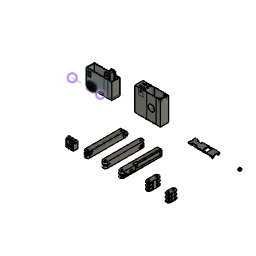
Table Lamp 2.0 v49 (Autodesk Fusion 360 design; units mm, degrees)
Autodesk Fusion 360 part; units mm, degrees
(part 1 of 2)
sketch "Schizzo1" plane through (0, 0, 0) normal (0, 0, 1) x (1, 0, 0)
  line L0 (0, 0) -> (100, 0)
  line L1 (100, 0) -> (100, 150)
  line L2 (100, 150) -> (0, 150)
  line L3 (0, 150) -> (0, 0)
  line L4 (199.5017, -0.6) -> (225.5017, -0.6)
  line L5 (225.5017, -0.6) -> (225.5017, 15.4)
  line L6 (225.5017, 15.4) -> (199.5017, 15.4)
  line L7 (199.5017, 15.4) -> (199.5017, -0.6)
  line L8 (212.5017, 15.4) -> (212.5017, -0.6) construction
  line L9 (199.5017, 7.4) -> (225.5017, 7.4) construction
  line L10 (199.5017, 15.4) -> (202.5017, 15.4)
  line L11 (202.5017, 15.4) -> (202.5017, -0.6)
  line L12 (202.5017, -0.6) -> (199.5017, -0.6)
  line L13 (199.5017, -0.6) -> (199.5017, 15.4)
  line L14 (212.5017, -0.6) -> (211.0017, -0.6)
  line L15 (211.0017, -0.6) -> (211.0017, 16)
  line L16 (211.0017, 16) -> (212.5017, 16)
  line L17 (212.5017, 16) -> (212.5017, -0.6)
  line L18 (222.5017, 15.4) -> (222.5017, -0.6)
  line L19 (214.0017, -0.6) -> (214.0017, 16)
  line L20 (199.5017, 12) -> (225.5017, 12) construction
  line L21 (207.0017, 18) -> (207.0017, -2) construction
  circle A0 centre (207.0017, 12) radius 1.6
  circle A1 centre (207.0017, 12) radius 3
  circle A2 centre (218.0017, 12) radius 3
  circle A3 centre (218.0017, 12) radius 1.6
  circle A4 centre (207.0017, 2.8) radius 3
  circle A5 centre (207.0017, 2.8) radius 1.6
  circle A6 centre (218.0017, 2.8) radius 1.6
  circle A7 centre (218.0017, 2.8) radius 3
  line L22 (100, 0) -> (84, 0) construction
  line L23 (84, 0) -> (84, 26) construction
  line L24 (84, 26) -> (100, 26) construction
  line L25 (100, 26) -> (100, 0) construction
  line L26 (107.0803, 18.5) -> (75, 18.5) construction
  line L27 (91.0401, 18.5) -> (91.0401, -5) construction
  line L28 (96.6, 35.1789) -> (96.6, -8.0692) construction
  line L29 (84, 13) -> (118.3318, 13) construction
  circle A8 centre (96.6, 18.5) radius 1.4
  circle A9 centre (85.4803, 18.5) radius 1.4
  circle A10 centre (96.6, 7.5) radius 1.4
  circle A11 centre (85.4803, 7.5) radius 1.4
  line L30 (259, 0) -> (275, 0)
  line L31 (275, 0) -> (275, 140)
  line L32 (275, 140) -> (259, 140)
  line L33 (259, 140) -> (259, 0)
  circle A12 centre (267, 8) radius 8
  circle A13 centre (267, 8) radius 3.1
  line L34 (466.5, 7.7189) -> (482.5, 7.7189)
  line L35 (482.5, 7.7189) -> (482.5, 51.7189)
  line L36 (482.5, 51.7189) -> (466.5, 51.7189)
  line L37 (466.5, 51.7189) -> (466.5, 7.7189)
  line L38 (474.5, 51.7189) -> (474.5, 7.7189) construction
  line L39 (466.5, 29.7189) -> (482.5, 29.7189) construction
  line L40 (459.1758, 43.7189) -> (505, 43.7189) construction
  line L41 (458.8216, 15.7189) -> (496.8919, 15.7189) construction
  circle A14 centre (474.5, 15.7189) radius 8
  circle A15 centre (474.5, 43.7189) radius 8
  circle A16 centre (474.5, 43.7189) radius 3.1
  circle A17 centre (474.5, 15.7189) radius 3.1
  line L42 (480, 33.5) -> (480, 25.9377) construction
  line L43 (482.5, 23.7189) -> (477.5, 23.7189)
  line L44 (477.5, 23.7189) -> (477.5, 35.7189)
  line L45 (477.5, 35.7189) -> (482.5, 35.7189)
  line L46 (482.5, 35.7189) -> (482.5, 23.7189)
  line L47 (482.5, 23.7189) -> (477.5, 35.7189) construction
  line L48 (477.5, 23.7189) -> (482.5, 35.7189) construction
  circle A18 centre (474.5, 43.7189) radius 8.5
  circle A19 centre (474.5, 15.7189) radius 8.5
  line L49 (243.0609, 253.7386) -> (303.0609, 253.7386)
  line L50 (303.0609, 253.7386) -> (303.0609, 226.7386)
  line L51 (303.0609, 226.7386) -> (243.0609, 226.7386)
  line L52 (243.0609, 226.7386) -> (243.0609, 253.7386)
  line L53 (244.2275, 240.2386) -> (345, 240.2386) construction
  line L54 (256.5609, 255) -> (256.5609, 215) construction
  circle A20 centre (256.5609, 240.2386) radius 13.5
  line L55 (273.0609, 253.7386) -> (273.0609, 220) construction
  line L56 (243.0609, 240.2386) -> (327.4169, 240.2386) construction
  circle A21 centre (289.5609, 240.2386) radius 13.5
  circle A22 centre (256.5609, 240.2386) radius 13.5
  circle A23 centre (289.5609, 240.2386) radius 13.5
  line L57 (241.0609, 254.7386) -> (305.0609, 254.7386)
  line L58 (305.0609, 254.7386) -> (305.0609, 225.7386)
  line L59 (305.0609, 225.7386) -> (241.0609, 225.7386)
  line L60 (241.0609, 225.7386) -> (241.0609, 254.7386)
  line L61 (321.5, 0) -> (337.5, 0)
  line L62 (337.5, 0) -> (337.5, 140)
  line L63 (337.5, 140) -> (321.5, 140)
  line L64 (321.5, 140) -> (321.5, 0)
  line L65 (329.5, 140) -> (329.5, 0) construction
  line L66 (321.5, 70) -> (342.446, 70) construction
  circle A24 centre (329.5, 8) radius 8
  circle A25 centre (329.5, 8) radius 3.1
  circle A26 centre (329.5, 132) radius 3.1
  circle A27 centre (329.5, 132) radius 8
  circle A28 centre (544.5, 32.4839) radius 8.5
  line L67 (536, 15.4839) -> (553, 15.4839) construction
  line L68 (552.5, 24.4839) -> (552.5, 23.4839)
  line L69 (536.5, 40.4839) -> (536.5, 7.4839)
  line L70 (544.5, 40.4839) -> (544.5, 7.4839) construction
  line L71 (536.5, 7.4839) -> (552.5, 7.4839)
  line L72 (547.5, 23.4839) -> (547.5, 24.4839)
  circle A29 centre (544.5, 32.4839) radius 3.1
  line L73 (552.5, 23.4839) -> (547.5, 23.4839)
  line L74 (552.5, 23.4839) -> (547.5, 24.4839) construction
  line L75 (536, 32.4839) -> (553, 32.4839) construction
  line L76 (536.5, 23.9839) -> (552.5, 23.9839) construction
  line L77 (552.5, 40.4839) -> (536.5, 40.4839)
  line L78 (552.5, 7.4839) -> (552.5, 40.4839)
  line L79 (550, 27.765) -> (550, 20.2027) construction
  circle A30 centre (544.5, 32.4839) radius 8
  line L80 (547.5, 23.4839) -> (552.5, 24.4839) construction
  circle A31 centre (544.5, 15.4839) radius 8
  circle A32 centre (544.5, 15.4839) radius 3.1
  circle A33 centre (544.5, 15.4839) radius 8.5
  line L81 (547.5, 24.4839) -> (552.5, 24.4839)
  line L82 (241.0609, 254.7386) -> (215.0609, 254.7386)
  line L83 (215.0609, 254.7386) -> (215.0609, 225.7386)
  line L84 (215.0609, 225.7386) -> (241.0609, 225.7386)
  line L85 (241.0609, 225.7386) -> (241.0609, 254.7386)
  line L86 (402.6629, 225.4895) -> (488.2629, 225.4895)
  line L87 (488.2629, 225.4895) -> (488.2629, 250.4895)
  line L88 (488.2629, 250.4895) -> (402.6629, 250.4895)
  line L89 (402.6629, 250.4895) -> (402.6629, 225.4895)
  line L90 (48.9231, 250) -> (138.9231, 250)
  line L91 (138.9231, 250) -> (138.9231, 221)
  line L92 (138.9231, 221) -> (48.9231, 221)
  line L93 (48.9231, 221) -> (48.9231, 250)
  line L94 (50.9231, 248) -> (136.9231, 248)
  line L95 (136.9231, 248) -> (136.9231, 223)
  line L96 (136.9231, 223) -> (50.9231, 223)
  line L97 (50.9231, 223) -> (50.9231, 248)
  line L98 (48.9231, 235.5) -> (138.9231, 235.5) construction
  line L99 (110.9231, 248) -> (124.9231, 248)
  line L100 (124.9231, 248) -> (124.9231, 243)
  line L101 (124.9231, 243) -> (110.9231, 243)
  line L102 (110.9231, 243) -> (110.9231, 248)
  line L103 (110.9231, 228) -> (110.9231, 223)
  line L104 (124.9231, 228) -> (110.9231, 228)
  line L105 (124.9231, 223) -> (124.9231, 228)
  line L106 (110.9231, 223) -> (124.9231, 223)
  line L107 (324, 0) -> (335, 140) construction
  line L108 (279.5609, 247.7386) -> (266.5609, 247.7386)
  line L109 (266.5609, 247.7386) -> (266.5609, 232.7386)
  line L110 (266.5609, 232.7386) -> (279.5609, 232.7386)
  line L111 (279.5609, 232.7386) -> (279.5609, 247.7386)
  line L112 (279.5609, 247.7386) -> (266.5609, 232.7386) construction
  line L113 (266.5609, 247.7386) -> (279.5609, 232.7386) construction
  line L114 (402.6629, 237.9895) -> (488.2629, 237.9895) construction
  line L115 (458.2629, 250.4895) -> (458.2629, 225.4895) construction
  line L116 (465.7629, 247.9895) -> (450.7629, 247.9895)
  line L117 (450.7629, 247.9895) -> (450.7629, 227.9895)
  line L118 (450.7629, 227.9895) -> (465.7629, 227.9895)
  line L119 (465.7629, 227.9895) -> (465.7629, 247.9895)
  line L120 (465.7629, 247.9895) -> (450.7629, 227.9895) construction
  line L121 (450.7629, 247.9895) -> (465.7629, 227.9895) construction
  line L122 (414.4629, 250.4895) -> (428.8629, 250.4895)
  line L123 (428.8629, 250.4895) -> (428.8629, 245.2895)
  line L124 (428.8629, 245.2895) -> (414.4629, 245.2895)
  line L125 (414.4629, 245.2895) -> (414.4629, 250.4895)
  line L126 (414.4629, 230.6895) -> (414.4629, 225.4895)
  line L127 (428.8629, 230.6895) -> (414.4629, 230.6895)
  line L128 (428.8629, 225.4895) -> (428.8629, 230.6895)
  line L129 (414.4629, 225.4895) -> (428.8629, 225.4895)
  line L130 (445.4629, 250.4895) -> (445.4629, 219.5723) construction
  line L131 (490.4629, 223.2895) -> (400.4629, 223.2895) construction
  line L132 (400.4629, 223.2895) -> (400.4629, 252.6895) construction
  line L133 (400.4629, 252.6895) -> (490.4629, 252.6895) construction
  line L134 (490.4629, 252.6895) -> (490.4629, 223.2895) construction
  line L135 (490.4629, 223.2895) -> (400.4629, 252.6895) construction
  line L136 (400.4629, 223.2895) -> (490.4629, 252.6895) construction
  line L137 (408.8629, 245.2895) -> (428.8629, 245.2895)
  line L138 (428.8629, 245.2895) -> (428.8629, 242.0895)
  line L139 (428.8629, 242.0895) -> (408.8629, 242.0895)
  line L140 (408.8629, 242.0895) -> (408.8629, 245.2895)
  line L141 (428.8629, 233.8895) -> (408.8629, 233.8895)
  line L142 (408.8629, 233.8895) -> (408.8629, 230.6895)
  line L143 (408.8629, 230.6895) -> (428.8629, 230.6895)
  line L144 (428.8629, 230.6895) -> (428.8629, 233.8895)
  line L145 (380, 0) -> (396, 0)
  line L146 (396, 0) -> (396, 140)
  line L147 (396, 140) -> (380, 140)
  line L148 (380, 140) -> (380, 0)
  line L149 (388, 140) -> (388, 0) construction
  circle A34 centre (388, 8) radius 8
  circle A35 centre (388, 8) radius 3
  line L150 (484.4629, 228.2895) -> (488.2629, 228.2895)
  line L151 (488.2629, 228.2895) -> (488.2629, 225.4895)
  line L152 (488.2629, 225.4895) -> (484.4629, 225.4895)
  line L153 (484.4629, 225.4895) -> (484.4629, 228.2895)
  line L154 (485.4629, 229.2895) -> (488.2629, 229.2895)
  line L155 (488.2629, 229.2895) -> (488.2629, 225.4895)
  line L156 (488.2629, 225.4895) -> (485.4629, 225.4895)
  line L157 (485.4629, 225.4895) -> (485.4629, 229.2895)
  line L158 (484.4629, 250.4895) -> (484.4629, 247.6895)
  line L159 (484.4629, 247.6895) -> (488.2629, 247.6895)
  line L160 (485.4629, 246.6895) -> (488.2629, 246.6895)
  line L161 (485.4629, 250.4895) -> (485.4629, 246.6895)
  line L162 (488.2629, 250.4895) -> (484.4629, 250.4895)
  line L163 (488.2629, 246.6895) -> (488.2629, 250.4895)
  circle A36 centre (575, 235) radius 3.1
  circle A37 centre (575, 235) radius 5
  line L164 (486.2629, 241.4895) -> (488.2629, 241.4895)
  line L165 (488.2629, 241.4895) -> (488.2629, 234.4895)
  line L166 (488.2629, 234.4895) -> (486.2629, 234.4895)
  line L167 (486.2629, 234.4895) -> (486.2629, 241.4895)
  line L168 (404.6629, 241.4895) -> (402.6629, 241.4895)
  line L169 (402.6629, 241.4895) -> (402.6629, 234.4895)
  line L170 (402.6629, 234.4895) -> (404.6629, 234.4895)
  line L171 (404.6629, 234.4895) -> (404.6629, 241.4895)
  line L172 (428.8629, 245.2895) -> (427.8629, 245.2895)
  line L173 (427.8629, 245.2895) -> (427.8629, 242.0895)
  line L174 (427.8629, 242.0895) -> (428.8629, 242.0895)
  line L175 (428.8629, 242.0895) -> (428.8629, 245.2895)
  line L176 (427.8629, 230.6895) -> (427.8629, 233.8895)
  line L177 (408.8629, 245.2895) -> (409.8629, 245.2895)
  line L178 (409.8629, 245.2895) -> (409.8629, 242.0895)
  line L179 (409.8629, 242.0895) -> (408.8629, 242.0895)
  line L180 (408.8629, 242.0895) -> (408.8629, 245.2895)
  line L181 (409.8629, 230.6895) -> (409.8629, 233.8895)
  line L182 (215.0017, 9.9) -> (210.0017, 9.9)
  line L183 (210.0017, 9.9) -> (210.0017, 4.9)
  line L184 (210.0017, 4.9) -> (215.0017, 4.9)
  line L185 (215.0017, 4.9) -> (215.0017, 9.9)
  line L186 (215.0017, 9.9) -> (210.0017, 4.9) construction
  line L187 (210.0017, 9.9) -> (215.0017, 4.9) construction
  line L188 (552.5, 29.6116) -> (536.5, 30) construction
  line L189 (552.5, 18.3561) -> (536.5, 18.3561) construction
  point P0 (480, 29.7189)
  point P1 (550, 23.9839)
  point P2 (273.0609, 240.2386)
  point P3 (212.5017, 7.4)
  point P4 (273.0609, 240.2386)
  point P5 (458.2629, 237.9895)
  point P6 (445.4629, 237.9895)
  point P7 (212.5017, 7.4)
  dimension "d1" = 100
  dimension "d2" = 150
  dimension "d3" = 26
  dimension "d4" = 16
  dimension "d5" = 3
  dimension "d6" = 1.5
  dimension "d17" = 3.4
  dimension "d18" = 7.5
  dimension "d19" = 3.2
  dimension "d20" = 6
  dimension "d27" = 16
  dimension "d28" = 26
  dimension "d29" = 7.5
  dimension "d30" = 3.4
  dimension "d31" = 2.8
  dimension "d34" = 16
  dimension "d35" = 140
  dimension "d36" = 8
  dimension "d37" = 6.2
  dimension "d69" = 16
  dimension "d70" = 44
  dimension "d71" = 8
  dimension "d72" = 8
  dimension "d73" = 16
  dimension "d74" = 16
  dimension "d75" = 6.2
  dimension "d76" = 6.2
  dimension "d89" = 5
  dimension "d93" = 17
  dimension "d94" = 17
  dimension "d95" = 60
  dimension "d96" = 27
  dimension "d97" = 13.5
  dimension "d98" = 13.5
  dimension "d104" = 16
  dimension "d105" = 140
  dimension "d106" = 16
  dimension "d107" = 6.2
  dimension "d120" = 16
  dimension "d121" = 33
  dimension "d122" = 8
  dimension "d123" = 8
  dimension "d124" = 16
  dimension "d125" = 16
  dimension "d126" = 6.2
  dimension "d127" = 6.2
  dimension "d128" = 5
  dimension "d129" = 17
  dimension "d130" = 17
  dimension "d150" = 90
  dimension "d157" = 64
  dimension "d158" = 29
  dimension "d160" = 25
  dimension "d196" = 2
  dimension "d197" = 90
  dimension "d198" = 29
  dimension "d199" = 2
  dimension "d200" = 2
  dimension "d201" = 2
  dimension "d202" = 2
  dimension "d222" = 14
  dimension "d223" = 5
  dimension "d226" = 14
  dimension "d261" = 2.5
  dimension "d262" = 2.5
  dimension "d357" = 13
  dimension "d358" = 15
  dimension "d361" = 30
  dimension "d362" = 15
  dimension "d363" = 20
  dimension "d364" = 14.4
  dimension "d365" = 5.2
  dimension "d366" = 11.8
  dimension "d377" = 90
  dimension "d379" = 2.2
  dimension "d380" = 2.2
  dimension "d381" = 20
  dimension "d382" = 3.2
  dimension "d391" = 16
  dimension "d392" = 140
  dimension "d393" = 16
  dimension "d400" = 6
  dimension "d431" = 3.8
  dimension "d432" = 2.8
  dimension "d433" = 2.8
  dimension "d434" = 3.8
  dimension "d442" = 6.2
  dimension "d443" = 10
  dimension "d446" = 2
  dimension "d447" = 7
  dimension "d471" = 1
  dimension "d472" = 1
  dimension "d473" = 5
  dimension "d474" = 5
  dimension "d476" = 28
  dimension "d481" = 11.2554
  constraint horizontal L0
  constraint vertical L1
  constraint horizontal L2
  constraint vertical L3
  constraint coincident L0.start L3.end
  constraint horizontal L4
  constraint vertical L5
  constraint horizontal L6
  constraint vertical L7
  constraint midpoint L6 L8.start
  constraint midpoint L4 L8.end
  constraint midpoint L7 L9.start
  constraint midpoint L5 L9.end
  constraint horizontal L10
  constraint vertical L11
  constraint horizontal L12
  constraint vertical L13
  constraint coincident L4 L11.end
  constraint horizontal L14
  constraint vertical L15
  constraint horizontal L16
  constraint vertical L17
  constraint symmetric L10.end L17 L18.start
  constraint symmetric L11.end L17 L18.end
  constraint symmetric L14.end L17 L19.start
  constraint symmetric L15.end L17 L19.end
  constraint perpendicular L13 L20
  constraint perpendicular L4 L21
  constraint coincident L21 A0.centre
  constraint coincident L20 A0.centre
  constraint concentric A0 A1
  constraint symmetric L8 A0 A3
  constraint symmetric L8 A1 A2
  constraint symmetric L9 A0 A5
  constraint symmetric L9 A1 A4
  constraint symmetric L9 A2 A7
  constraint symmetric L9 A3 A6
  constraint horizontal L22
  constraint vertical L23
  constraint horizontal L24
  constraint vertical L25
  constraint perpendicular L1 L26
  constraint midpoint L26 L27.start
  constraint perpendicular L22 L27
  constraint perpendicular L0 L28
  constraint midpoint L23 L29.start
  constraint perpendicular L25 L29
  constraint coincident L26 A8.centre
  constraint coincident L28 A8.centre
  constraint symmetric L27 A8 A9
  constraint symmetric L29 A8 A10
  constraint symmetric L29 A9 A11
  constraint horizontal L30
  constraint vertical L31
  constraint horizontal L32
  constraint vertical L33
  constraint tangent L33 A12
  constraint tangent L30 A12
  constraint concentric A12 A13
  constraint horizontal L34
  constraint vertical L35
  constraint horizontal L36
  constraint vertical L37
  constraint midpoint L36 L38.start
  constraint midpoint L34 L38.end
  constraint midpoint L37 L39.start
  constraint midpoint L35 L39.end
  constraint perpendicular L35 L40
  constraint perpendicular L35 L41
  constraint coincident L41 A14.centre
  constraint coincident L38 A14.centre
  constraint coincident L38 A15.centre
  constraint coincident L40 A15.centre
  constraint concentric A15 A16
  constraint concentric A14 A17
  constraint parallel L38 L42
  constraint horizontal L43
  constraint perpendicular L43 L44
  constraint parallel L43 L45
  constraint parallel L44 L46
  constraint coincident L47 P0
  constraint coincident L48 P0
  constraint midpoint L42 P0
  constraint tangent A15 L45
  constraint tangent A14 L43
  constraint collinear L35 L46
  constraint concentric A16 A18
  constraint concentric A17 A19
  constraint horizontal L49
  constraint vertical L50
  constraint horizontal L51
  constraint vertical L52
  constraint perpendicular L50 L53
  constraint perpendicular L49 L54
  constraint coincident L54 A20.centre
  constraint coincident L53 A20.centre
  constraint midpoint L49 L55.start
  constraint perpendicular L49 L55
  constraint midpoint L52 L56.start
  constraint perpendicular L52 L56
  constraint symmetric A20 L55 A21
  constraint symmetric A20 L56 A22
  constraint symmetric L56 A21 A23
  constraint tangent L49 A20
  constraint horizontal L61
  constraint vertical L62
  constraint horizontal L63
  constraint vertical L64
  constraint midpoint L63 L65.start
  constraint midpoint L61 L65.end
  constraint midpoint L64 L66.start
  constraint perpendicular L62 L66
  constraint coincident L65 A24.centre
  constraint tangent L61 A24
  constraint concentric A24 A25
  constraint symmetric L66 A24 A27
  constraint symmetric L66 A25 A26
  constraint horizontal L71
  constraint vertical L78
  constraint horizontal L77
  constraint vertical L69
  constraint midpoint L70.start L77
  constraint midpoint L70.end L71
  constraint midpoint L76.start L69
  constraint midpoint L76.end L78
  constraint perpendicular L75 L78
  constraint perpendicular L67 L78
  constraint coincident A31.centre L67
  constraint coincident A31.centre L70
  constraint coincident A28.centre L70
  constraint coincident A28.centre L75
  constraint concentric A29 A30
  constraint concentric A31 A32
  constraint parallel L70 L79
  constraint horizontal L73
  constraint perpendicular L72 L73
  constraint parallel L73 L81
  constraint parallel L68 L72
  constraint coincident P1 L74
  constraint coincident P1 L80
  constraint midpoint P1 L79
  constraint tangent A30 L81
  constraint tangent L73 A31
  constraint collinear L68 L78
  constraint concentric A28 A29
  constraint concentric A32 A33
  constraint horizontal L82
  constraint vertical L83
  constraint horizontal L84
  constraint vertical L85
  constraint coincident L57.start L60.end
  constraint coincident L59.end L60.start
  constraint vertical L87
  constraint vertical L89
  constraint coincident L55 P4
  constraint coincident L53 P4
  constraint horizontal L90
  constraint vertical L91
  constraint horizontal L92
  constraint vertical L93
  constraint horizontal L94
  constraint vertical L95
  constraint horizontal L96
  constraint vertical L97
  constraint midpoint L93 L98.start
  constraint midpoint L91 L98.end
  constraint horizontal L99
  constraint vertical L100
  constraint horizontal L101
  constraint vertical L102
  constraint collinear L94 L99
  constraint symmetric L98 L99.start L103.end
  constraint symmetric L98 L99.end L105.start
  constraint symmetric L98 L100.end L104.start
  constraint symmetric L98 L101.end L103.start
  constraint coincident L61 L107.start
  constraint coincident L63 L107.end
  constraint midpoint L9 P7
  constraint horizontal L108
  constraint perpendicular L108 L109
  constraint parallel L108 L110
  constraint parallel L109 L111
  constraint coincident L112 P4
  constraint coincident L113 P4
  constraint coincident P4 P2
  constraint midpoint L89 L114.start
  constraint midpoint L87 L114.end
  constraint coincident L88 L115.start
  constraint coincident L86 L115.end
  constraint perpendicular L86 L115
  constraint horizontal L116
  constraint perpendicular L116 L117
  constraint parallel L116 L118
  constraint parallel L117 L119
  constraint coincident L120 P5
  constraint coincident L121 P5
  constraint midpoint L115 P5
  constraint perpendicular L87 L88
  constraint horizontal L122
  constraint vertical L123
  constraint horizontal L124
  constraint vertical L125
  constraint symmetric L114 L122.start L126.end
  constraint symmetric L114 L122.end L128.start
  constraint symmetric L114 L123.end L127.start
  constraint symmetric L114 L124.end L126.start
  constraint collinear L88 L122
  constraint midpoint L88 L130.start
  constraint perpendicular L88 L130
  constraint horizontal L131
  constraint perpendicular L131 L132
  constraint parallel L131 L133
  constraint parallel L132 L134
  constraint coincident L135 P6
  constraint coincident L136 P6
  constraint midpoint L114 P6
  constraint horizontal L137
  constraint vertical L138
  constraint horizontal L139
  constraint vertical L140
  constraint coincident L123.end L124.start
  constraint symmetric L114 L137.start L142.end
  constraint symmetric L114 L138.end L141.start
  constraint symmetric L114 L139.end L141.end
  constraint horizontal L145
  constraint vertical L146
  constraint horizontal L147
  constraint vertical L148
  constraint midpoint L147 L149.start
  constraint midpoint L145 L149.end
  constraint coincident L149 A34.centre
  constraint tangent L145 A34
  constraint concentric A34 A35
  constraint horizontal L150
  constraint vertical L151
  constraint horizontal L152
  constraint vertical L153
  constraint horizontal L154
  constraint vertical L155
  constraint horizontal L156
  constraint vertical L157
  constraint coincident L86.end L87.start L2.end
  constraint coincident L86.end L87.start
  constraint symmetric L114 L150.start L158.end
  constraint symmetric L114 L150.end L159.end
  constraint symmetric L114 L86.end L87.end
  constraint symmetric L114 L152.end L158.start
  constraint symmetric L114 L154.start L160.start
  constraint symmetric L114 L154.end L160.end
  constraint symmetric L114 L156.end L161.start
  constraint concentric A36 A37
  constraint horizontal L164
  constraint vertical L165
  constraint horizontal L166
  constraint vertical L167
  constraint midpoint L114.end L165
  constraint symmetric L130 L164.start L168.start
  constraint symmetric L130 L164.end L168.end
  constraint symmetric L130 L165.end L169.end
  constraint symmetric L130 L166.end L170.end
  constraint horizontal L172
  constraint vertical L173
  constraint horizontal L174
  constraint vertical L175
  constraint coincident L139 L173.end
  constraint symmetric L114 L172.end L176.start
  constraint symmetric L114 L173.end L176.end
  constraint horizontal L177
  constraint vertical L178
  constraint horizontal L179
  constraint vertical L180
  constraint symmetric L114 L177.end L181.start
  constraint symmetric L114 L178.end L181.end
  constraint collinear L139 L179
  constraint horizontal L182
  constraint perpendicular L182 L183
  constraint parallel L182 L184
  constraint parallel L183 L185
  constraint coincident L186 P7
  constraint coincident L187 P7
  constraint coincident P7 P3
  constraint coincident L5 L20.end
  constraint coincident L7 L20.start
  constraint coincident L75.end A28
  constraint coincident L67.end A33
  constraint coincident L67.start A33
  constraint coincident L75.start A28
  constraint coincident L78 L188.start
  constraint coincident A28 L188.start
  constraint coincident L69 L188.end
  constraint coincident A33 L189.start
  constraint coincident L78 L189.start
  constraint coincident A33 L189.end
  constraint coincident L69 L189.end
  measures "d1" distance of L0.start L0.end
  measures "d2" distance of L0.start L2.end
  measures "d3" distance of L4.start L4.end
  measures "d4" distance of L4.start L6.end
  measures "d5" distance of L6.end L10.end
  measures "d6" distance of L8.end L14.end
  measures "d17" distance of L6 L20
  measures "d18" distance of L13 L21
  measures "d19" diameter of A0
  measures "d20" diameter of A1
  measures "d27" distance of L0.end L22.end
  measures "d28" distance of L0.end L24.end
  measures "d29" distance of L24 L26
  measures "d30" distance of L1 L28
  measures "d31" diameter of A8
  measures "d34" distance of L31 L33
  measures "d35" distance of L30 L32
  measures "d36" radius of A12
  measures "d37" diameter of A13
  measures "d69" distance of L34.start L34.end
  measures "d70" distance of L34.start L36.end
  measures "d71" distance of L36 L40
  measures "d72" distance of L34 L41
  measures "d73" diameter of A14
  measures "d74" diameter of A15
  measures "d75" diameter of A16
  measures "d76" diameter of A17
  measures "d89" distance of L44.end L45.end
  measures "d93" diameter of A18
  measures "d94" diameter of A19
  measures "d95" distance of L49.start L49.end
  measures "d96" distance of L49.start L51.end
  measures "d97" distance of L49 L53
  measures "d98" distance of L52 L54
  measures "d104" distance of L61.start L61.end
  measures "d105" distance of L61.start L63.end
  measures "d106" diameter of A24
  measures "d107" diameter of A25
  measures "d120" distance of L69.end L71.end
  measures "d121" distance of L69.start L69.end
  measures "d122" distance of L75 L77
  measures "d123" distance of L67 L71
  measures "d124" diameter of A31
  measures "d125" diameter of A30
  measures "d126" diameter of A29
  measures "d127" diameter of A32
  measures "d128" distance of L72.end L68.start
  measures "d129" diameter of A28
  measures "d130" diameter of A33
  measures "d150" distance of L58 L83
  measures "d157" distance of L58 L85
  measures "d158" distance of L57 L59
  measures "d160" distance of L86.start L88.end
  measures "d196" distance of L52 L85
  measures "d197" distance of L90.start L90.end
  measures "d198" distance of L90.start L92.end
  measures "d199" distance of L93 L97
  measures "d200" distance of L92 L96
  measures "d201" distance of L91 L95
  measures "d202" distance of L90 L94
  measures "d222" distance of L100 L102
  measures "d223" distance of L99 L101
  measures "d226" distance of L91 L100
  measures "d261" distance of L64 L107.start
  measures "d262" distance of L62 L107.end
  measures "d357" distance of L109.end L110.end
  measures "d358" distance of L108.end L109.end
  measures "d361" distance of L87 L115
  measures "d362" distance of L117.end L118.end
  measures "d363" distance of L116.end L117.end
  measures "d364" distance of L122.start L122.end
  measures "d365" distance of L122.start L124.end
  measures "d366" distance of L89 L125
  measures "d377" distance of L132.end L133.end
  measures "d379" distance of L89 L132
  measures "d380" distance of L88 L133
  measures "d381" distance of L137.start L123.end
  measures "d382" distance of L137.start L139.end
  measures "d391" distance of L145.start L145.end
  measures "d392" distance of L145.start L147.end
  measures "d393" diameter of A34
  measures "d400" diameter of A35
  measures "d431" distance of L150.start L150.end
  measures "d432" distance of L150.start L152.end
  measures "d433" distance of L154.start L154.end
  measures "d434" distance of L154.start L156.end
  measures "d442" diameter of A36
  measures "d443" diameter of A37
  measures "d446" distance of L164.start L164.end
  measures "d447" distance of L164.start L166.end
  measures "d471" distance of L123.end L172.end
  measures "d472" distance of L137.start L177.end
  measures "d473" distance of L183.end L184.end
  measures "d474" distance of L182.end L183.end
  measures "d476" distance of L40 L41
  measures "d481" distance of L188.start L189.start
extrude "Estrusione1" add sketch "Schizzo1" along normal blind 29 contours L4 L6 L7 L10 L11 L12 L13 | L4 L14 L15 L17 L184 | L4 L17 L19 L184 | L15 L17 L182 L184 | L6 L15 L17 L182 | L17 L19 L182 L184 | L6 L17 L19 L182 | L4 L5 L6 L18 makes body 1 at (199.5017, 10.0667, 9.6667) makes body 2 at (211.0017, 4.7333, 9.6667) makes body 3 at (222.5017, 10.0667, 9.6667)
extrude "Estrusione2" add sketch "Schizzo1" along normal blind 6 contours L4 L6 L11 L15 L182 L183 L184 | L15 L182 L183 L184 | L4 L6 L18 L19 L182 L184 L185 | L19 L182 L184 L185 | A0 | A1 | A2 | A3 | A4 | A5 | A6 | A7 bodies 1 2 3
extrude "Estrusione5" cut sketch "Schizzo1" along normal blind 6 contours A0 | A3 | A5 | A6 bodies 1
extrude "Estrusione6" cut sketch "Schizzo1" along normal blind 6 and the other way blind -2.5 contours A1 | A2 | A4 | A7 bodies 1
extrude "Estrusione67" cut sketch "Schizzo1" along normal blind 14 contours L15 L182 L183 L184 | L15 L17 L182 L184 | L17 L19 L182 L184 | L19 L182 L184 L185 bodies 1
sketch "Schizzo2" plane through (225.5017, 0, 0) normal (1, 0, 0) x (0, 1, 0)
  line L0 (-0.6, 0) -> (15.4, 0)
  line L1 (15.4, 0) -> (15.4, 29)
  line L2 (15.4, 29) -> (-0.6, 29)
  line L3 (-0.6, 29) -> (-0.6, 0)
  line L4 (7.4, 29) -> (7.4, -6) construction
  line L5 (-10.0406, 21) -> (18.9594, 21) construction
  circle A0 centre (7.4, 21) radius 8
  circle A1 centre (7.4, 21) radius 3.1
  dimension "d11" = 8
  dimension "d12" = 6.2
  dimension "d478" = 16
  constraint midpoint L2 L4.start
  constraint perpendicular L2 L4
  constraint perpendicular L1 L5
  constraint coincident L4 A0.centre
  constraint coincident L5 A0.centre
  constraint coincident L4.start A0
  constraint concentric A0 A1
  measures "d11" distance of L2 L5
  measures "d12" diameter of A1
  measures "d478" diameter of A0
extrude "Estrusione3" cut sketch "Schizzo2" against normal blind 26 contours L2 L3 A0 | L1 L2 A0 bodies 1
extrude "Estrusione4" cut sketch "Schizzo2" against normal blind 26 contours A1 bodies 1
extrude "Estrusione8" add sketch "Schizzo1" along normal blind 20 separate body contours L30 L33 A12 | L30 L31 A12 | A12 | L31 L32 L33 A12 makes body 4
sketch "Schizzo5" plane through (0, 0, 0) normal (0, -1, 0) x (1, 0, 0)
  line L0 (259, 0) -> (275, 0)
  line L1 (275, 0) -> (275, 20)
  line L2 (275, 20) -> (259, 20)
  line L3 (259, 20) -> (259, 0)
  line L4 (267, 20) -> (267, 0) construction
  line L5 (259, 10) -> (275, 10) construction
  line L6 (275, 11.5) -> (259, 11.5)
  line L7 (259, 11.5) -> (259, 8.5)
  line L8 (259, 8.5) -> (275, 8.5)
  line L9 (275, 8.5) -> (275, 11.5)
  line L10 (275, 11.5) -> (259, 8.5) construction
  line L11 (259, 11.5) -> (275, 8.5) construction
  line L12 (269.5, 0) -> (264.5, 0)
  line L13 (264.5, 0) -> (264.5, 20)
  line L14 (264.5, 20) -> (269.5, 20)
  line L15 (269.5, 20) -> (269.5, 0)
  line L16 (269.5, 0) -> (264.5, 20) construction
  line L17 (264.5, 0) -> (269.5, 20) construction
  line L18 (269.5, 17.25) -> (272.5, 17.25)
  line L19 (272.5, 17.25) -> (272.5, 13.25)
  line L20 (272.5, 13.25) -> (269.5, 13.25)
  line L21 (269.5, 13.25) -> (269.5, 17.25)
  line L22 (269.5, 17.2244) -> (275, 17.2244)
  line L23 (275, 17.2244) -> (275, 13.2244)
  line L24 (275, 13.2244) -> (269.5, 13.2244)
  line L25 (269.5, 13.2244) -> (269.5, 17.2244)
  point P0 (267, 10)
  point P1 (267, 10)
  dimension "d63" = 16
  dimension "d64" = 3
  dimension "d141" = 5
  dimension "d142" = 20
  dimension "d301" = 3
  dimension "d302" = 4
  dimension "d305" = 2.75
  dimension "d306" = 2.5
  dimension "d307" = 5.5
  constraint midpoint L2 L4.start
  constraint midpoint L0 L4.end
  constraint midpoint L3 L5.start
  constraint midpoint L1 L5.end
  constraint horizontal L6
  constraint perpendicular L6 L7
  constraint parallel L6 L8
  constraint parallel L7 L9
  constraint coincident L10 P1
  constraint coincident L11 P1
  constraint midpoint L5 P1
  constraint horizontal L12
  constraint perpendicular L12 L13
  constraint parallel L12 L14
  constraint parallel L13 L15
  constraint coincident L16 P1
  constraint coincident L17 P1
  constraint coincident P1 P0
  constraint horizontal L18
  constraint vertical L19
  constraint horizontal L20
  constraint vertical L21
  constraint horizontal L22
  constraint vertical L23
  constraint horizontal L24
  constraint vertical L25
  constraint collinear L1 L23
  measures "d63" distance of L7.end L8.end
  measures "d64" distance of L6.end L7.end
  measures "d141" distance of L13.end L14.end
  measures "d142" distance of L12.end L13.end
  measures "d301" distance of L18.start L18.end
  measures "d302" distance of L18.start L20.end
  measures "d305" distance of L2 L18
  measures "d306" distance of L1 L19
  measures "d307" distance of L22.start L22.end
extrude "Estrusione16" cut sketch "Schizzo5" against normal blind 16.5 contours L3 L6 L7 L8 L13 | L6 L8 L13 L15 | L1 L6 L8 L9 L15 bodies 4
extrude "Estrusione17" cut sketch "Schizzo1" along normal blind 20 contours L30 L33 A12 | L30 L31 A12 bodies 4
extrude "Estrusione32" cut sketch "Schizzo5" against normal blind 0.2 contours L0 L8 L12 L13 L15 | L2 L6 L13 L14 L15 L21 L25 bodies 4
sketch "Schizzo3" plane through (275, 0, 0) normal (1, 0, 0) x (0, 1, 0)
  line L0 (8, 0) -> (140, 0)
  line L1 (140, 0) -> (140, 20)
  line L2 (140, 20) -> (8, 20)
  line L3 (140, 10) -> (-20, 10) construction
  circle A0 centre (132, 10) radius 8
  line L4 (132, 20) -> (132, 0)
  circle A1 centre (132, 10) radius 3.1
  line L5 (8, 11.5) -> (16.5, 11.5)
  line L6 (16.5, 11.5) -> (16.5, 8.5)
  line L7 (16.5, 8.5) -> (8, 8.5)
  line L8 (8, 20) -> (8, 11.5)
  line L9 (8, 8.5) -> (8, 0)
  point P0 (0.2, 20)
  dimension "d43" = 16
  dimension "d54" = 6.2
  dimension "d479" = 20
  dimension "d480" = 139.8
  constraint midpoint L1 L3.start
  constraint perpendicular L1 L3
  constraint coincident L3 A0.centre
  constraint coincident L2 L4.start
  constraint coincident L0 L4.end
  constraint perpendicular L0 L4
  constraint concentric A0 A1
  constraint coincident L4 A0.centre
  measures "d43" diameter of A0
  measures "d54" diameter of A1
  measures "d479" distance of L0 L2
  measures "d480" distance of L1.end P0
sketch "Schizzo4" plane through (0, 140, 0) normal (0, 1, 0) x (-1, 0, 0)
  line L0 (-275, 0) -> (-259, 0)
  line L1 (-259, 0) -> (-259, 20)
  line L2 (-259, 20) -> (-275, 20)
  line L3 (-275, 20) -> (-275, 0)
  line L4 (-267, 20) -> (-267, 0) construction
  line L5 (-275, 10) -> (-259, 10) construction
  line L6 (-265.5, 20) -> (-268.5, 20)
  line L7 (-268.5, 20) -> (-268.5, 0)
  line L8 (-268.5, 0) -> (-265.5, 0)
  line L9 (-265.5, 0) -> (-265.5, 20)
  line L10 (-265.5, 20) -> (-268.5, 0) construction
  line L11 (-268.5, 20) -> (-265.5, 0) construction
  point P0 (-267, 10)
  dimension "d59" = 3
  dimension "d60" = 20
  constraint midpoint L2 L4.start
  constraint midpoint L0 L4.end
  constraint midpoint L3 L5.start
  constraint midpoint L1 L5.end
  constraint horizontal L6
  constraint perpendicular L6 L7
  constraint parallel L6 L8
  constraint parallel L7 L9
  constraint coincident L10 P0
  constraint coincident L11 P0
  constraint midpoint L4 P0
  measures "d59" distance of L7.end L8.end
  measures "d60" distance of L6.end L7.end
extrude "Estrusione15" cut sketch "Schizzo4" against normal blind 16.5 contours L0 L2 L6 L7 L8 L9 bodies 4
extrude "Estrusione10" cut sketch "Schizzo3" against normal blind 16 contours L0 L1 A0 L4 | L1 L2 A0 L4 bodies 4
extrude "Estrusione11" add sketch "Schizzo3" along normal blind 2 contours A0 L4 A1 | A0 L4 A1 | L4 A1 | L4 A1 bodies 4
extrude "Estrusione12" add 1 faces at (277, 130.2681, 12.3094) along direction (-1, 0, 0) blind 20 on bodies 4 bodies 4
extrude "Estrusione13" cut 1 faces at (277, 130.2681, 12.3094) along direction (-1, 0, 0) blind 3 from surface at 8.5 on bodies 4 bodies 4
extrude "Estrusione14" cut sketch "Schizzo3" along normal blind 2 and the other way blind 19 contours L4 A1 | L4 A1 bodies 4
ref_plane "Piano di lavoro2" through (269.5, 70, 10) normal (1, 0, 0) x (0, 1, 0)
sketch "Schizzo17" plane through (269.5, 0, 0) normal (1, 0, 0) x (0, 1, 0)
  line L0 (140, 20) -> (8, 20) construction
  line L1 (8, 0) -> (140, 0) construction
  line L2 (0, 17.25) -> (0, 13.25)
  line L3 (0, 17.25) -> (140, 17.25)
  line L4 (0, 13.25) -> (140, 13.25)
  line L5 (140, 13.25) -> (140, 17.25)
  constraint perpendicular L2 L3
  constraint perpendicular L2 L4
  constraint perpendicular L3 L5
extrude "Estrusione66" cut sketch "Schizzo17" along normal blind 3 bodies 4
extrude "Estrusione18" add sketch "Schizzo1" along normal blind 3 separate body contours A14 | L35 L37 A14 A19 | L35 L37 L43 L44 L45 A18 A19 | L35 L37 A15 A18 | A15 | L35 L43 L44 L45 L46 makes body 5
extrude "Estrusione20" add 1 faces at (477.0122, 31.7189, 3) along direction (0, 0, 1) blind 3 from surface at 8.5 on bodies 5 bodies 5 makes body 6
extrude "Estrusione21" add 1 faces at (477.0122, 31.7189, 14.5) along direction (0, 0, 1) blind 3 from surface at 8.5 on bodies 6 bodies 6 makes body 7
extrude "Estrusione22" add sketch "Schizzo1" along normal blind 26 contours L35 L43 L44 L45 L46 bodies 5 6 7
extrude "Estrusione24" add sketch "Schizzo1" along normal blind 20 separate body contours L61 L64 A24 | L61 L62 A24 | A24 | L62 L64 A24 A27 | L63 L64 A27 | A27 | L62 L63 A27 makes body 8
ref_plane "Piano di lavoro1" through (329.5, 70, 0) normal (0.996927, -0.07833, 0) x (0.07833, 0.996927, 0)
extrude "Estrusione65" cut sketch "Schizzo5" against normal blind 17 contours L1 L15 L19 L20 L22 L23 L24 L25 | L15 L19 L20 L21 L22 L25 bodies 4
sketch "Schizzo16" plane through (322.0121, -25.3009, 0) normal (0.996927, -0.07833, 0) x (0.07833, 0.996927, 0)
  line L0 (26.4364, 0) -> (166.0062, 0) construction
  line L1 (25.1831, 20) -> (166.0062, 20) construction
  line L2 (166.0062, 20) -> (166.0062, 0) construction
  line L3 (166.0062, 0) -> (25.1831, 0)
  line L4 (25.1831, 0) -> (25.1831, 20) construction
  line L5 (25.1831, 10) -> (166.0062, 10) construction
  line L6 (95.5947, 20) -> (95.5947, 0) construction
  line L7 (10.9048, 17.25) -> (25.1831, 17.25) construction
  line L8 (166.0062, 2.75) -> (175, 2.75) construction
  line L9 (25.1831, 14.25) -> (10, 14.25) construction
  line L10 (166.0062, 5.75) -> (175, 5.75) construction
  line L11 (25.1831, 17.25) -> (166.0062, 5.75)
  line L12 (166.0062, 5.75) -> (166.0062, 2.75)
  line L13 (166.0062, 2.75) -> (25.1831, 14.25)
  line L14 (25.1831, 14.25) -> (25.1831, 17.25)
  point P0 (25.1831, 20)
  dimension "d283" = 2.75
  dimension "d284" = 2.75
  dimension "d285" = 3
  dimension "d286" = 3
  constraint horizontal L1
  constraint vertical L2
  constraint horizontal L3
  constraint vertical L4
  constraint coincident L0.end L2.end
  constraint coincident P0 L1.start
  constraint midpoint L4 L5.start
  constraint midpoint L2 L5.end
  constraint midpoint L1 L6.start
  constraint midpoint L3 L6.end
  constraint coincident L4 L7.end
  constraint perpendicular L4 L7
  constraint coincident L2 L8.start
  constraint perpendicular L2 L8
  constraint coincident L4 L9.start
  constraint perpendicular L4 L9
  constraint coincident L2 L10.start
  constraint perpendicular L2 L10
  measures "d283" distance of L1 L7
  measures "d284" distance of L0 L8
  measures "d285" distance of L7 L9
  measures "d286" distance of L8 L10
extrude "Estrusione60" cut sketch "Schizzo16" along normal mid plane 4 bodies 8
sketch "Schizzo6" plane through (0, 0, 0) normal (0, -1, 0) x (1, 0, 0)
  line L0 (321.5, 0) -> (337.5, 0)
  line L1 (337.5, 0) -> (337.5, 20)
  line L2 (337.5, 20) -> (321.5, 20)
  line L3 (321.5, 20) -> (321.5, 0)
  line L4 (329.5, 20) -> (329.5, 0) construction
  line L5 (321.5, 10) -> (337.5, 10) construction
  line L6 (337.5, 8.5) -> (321.5, 8.5)
  line L7 (321.5, 8.5) -> (321.5, 11.5)
  line L8 (321.5, 11.5) -> (337.5, 11.5)
  line L9 (337.5, 11.5) -> (337.5, 8.5)
  line L10 (337.5, 8.5) -> (321.5, 11.5) construction
  line L11 (321.5, 8.5) -> (337.5, 11.5) construction
  line L12 (321.9938, 14.2468) -> (321.9938, 17.2468)
  line L13 (321.9938, 17.2468) -> (326.0062, 17.2212)
  line L14 (326.0062, 17.2212) -> (326.0062, 14.2212)
  line L15 (326.0062, 14.2212) -> (321.9938, 14.2468)
  line L16 (321.9938, 17.2468) -> (326.0062, 17.2468)
  line L17 (326.0062, 17.2468) -> (326.0062, 14.2212)
  line L18 (326.0062, 14.2212) -> (321.9938, 14.2212)
  line L19 (321.9938, 14.2212) -> (321.9938, 17.2468)
  line L20 (321.5, 17.2488) -> (326, 17.2488)
  line L21 (326, 17.2488) -> (326, 13.2488)
  line L22 (326, 13.2488) -> (321.5, 13.2488)
  line L23 (321.5, 13.2488) -> (321.5, 17.2488)
  point P0 (329.5, 10)
  dimension "d110" = 16
  dimension "d111" = 3
  dimension "d289" = 4.5
  dimension "d290" = 4
  constraint midpoint L2 L4.start
  constraint perpendicular L2 L4
  constraint midpoint L3 L5.start
  constraint midpoint L1 L5.end
  constraint horizontal L6
  constraint perpendicular L6 L7
  constraint parallel L6 L8
  constraint parallel L7 L9
  constraint coincident L10 P0
  constraint coincident L11 P0
  constraint midpoint L4 P0
  constraint horizontal L16
  constraint vertical L17
  constraint horizontal L18
  constraint vertical L19
  constraint coincident L14.end L15.start
  constraint coincident L12.end L13.start
  constraint horizontal L20
  constraint vertical L21
  constraint horizontal L22
  constraint vertical L23
  constraint collinear L3 L23
  measures "d110" distance of L7.end L8.end
  measures "d111" distance of L6.end L7.end
  measures "d289" distance of L20.start L20.end
  measures "d290" distance of L20.start L22.end
extrude "Estrusione61" cut sketch "Schizzo6" against normal blind 3 contours L3 L12 L18 L19 L20 L21 L22 L23 | L12 L13 L15 L19 L21 | L13 L16 L20 L21 | L15 L18 L19 bodies 8
extrude "Estrusione63" cut sketch "Schizzo6" against normal blind 17 contours L3 L12 L16 L18 L19 L20 L21 L22 L23 | L15 L18 L19 | L12 L13 L15 L19 L21 bodies 8
extrude "Estrusione25" cut sketch "Schizzo6" against normal blind 16.5 contours L1 L3 L6 L7 L8 L9 bodies 8
sketch "Schizzo7" plane through (0, 140, 0) normal (0, 1, 0) x (-1, 0, 0)
  line L0 (-337.5, 0) -> (-321.5, 0)
  line L1 (-321.5, 0) -> (-321.5, 20)
  line L2 (-321.5, 20) -> (-337.5, 20)
  line L3 (-337.5, 20) -> (-337.5, 0)
  line L4 (-329.5, 20) -> (-329.5, 0) construction
  line L5 (-337.5, 10) -> (-321.5, 10) construction
  line L6 (-321.5, 8.5) -> (-337.5, 8.5)
  line L7 (-337.5, 8.5) -> (-337.5, 11.5)
  line L8 (-337.5, 11.5) -> (-321.5, 11.5)
  line L9 (-321.5, 11.5) -> (-321.5, 8.5)
  line L10 (-321.5, 8.5) -> (-337.5, 11.5) construction
  line L11 (-337.5, 8.5) -> (-321.5, 11.5) construction
  line L12 (-332.9938, 5.7788) -> (-332.9938, 2.7788)
  line L13 (-332.9938, 2.7788) -> (-337.0062, 2.7532)
  line L14 (-337.0062, 2.7532) -> (-337.0062, 5.7532)
  line L15 (-337.0062, 5.7532) -> (-332.9938, 5.7788)
  line L16 (-337.5, 6.7579) -> (-333, 6.7579)
  line L17 (-333, 6.7579) -> (-333, 2.7579)
  line L18 (-333, 2.7579) -> (-337.5, 2.7579)
  line L19 (-337.5, 2.7579) -> (-337.5, 6.7579)
  point P0 (-329.5, 10)
  dimension "d114" = 16
  dimension "d115" = 3
  dimension "d293" = 4.5
  dimension "d294" = 4
  constraint midpoint L2 L4.start
  constraint midpoint L0 L4.end
  constraint midpoint L3 L5.start
  constraint midpoint L1 L5.end
  constraint horizontal L6
  constraint perpendicular L6 L7
  constraint parallel L6 L8
  constraint parallel L7 L9
  constraint coincident L10 P0
  constraint coincident L11 P0
  constraint midpoint L5 P0
  constraint horizontal L16
  constraint vertical L17
  constraint horizontal L18
  constraint vertical L19
  constraint collinear L3 L19
  measures "d114" distance of L7.end L8.end
  measures "d115" distance of L6.end L7.end
  measures "d293" distance of L16.start L16.end
  measures "d294" distance of L16.start L18.end
extrude "Estrusione62" cut sketch "Schizzo7" against normal blind 17 contours L3 L14 L15 L16 L17 L18 L19 | L13 L14 L15 L17 L18 | L13 L17 L18 bodies 8
extrude "Estrusione26" cut sketch "Schizzo7" against normal blind 16.5 contours L1 L3 L6 L7 L8 L9 bodies 8
extrude "Estrusione27" cut sketch "Schizzo1" along normal blind 20 contours L61 L64 A24 | L61 L62 A24 | L63 L64 A27 | L62 L63 A27 bodies 8
extrude "Estrusione28" add sketch "Schizzo1" along normal blind 3 separate body contours A28 L72 L73 L78 A33 L81 | A28 L69 L78 A30 | A30 | A28 L69 A33 | L69 L78 A31 A33 | L68 L72 L73 L78 L81 | A31 makes body 9
extrude "Estrusione29" add 1 faces at (547.6265, 24.1505, 3) along direction (0, 0, 1) blind 3 from surface at 8.5 on bodies 9 bodies 9 makes body 10
extrude "Estrusione30" add 1 faces at (547.6265, 24.1505, 14.5) along direction (0, 0, 1) blind 3 from surface at 8.5 on bodies 10 bodies 10 makes body 11
extrude "Estrusione31" add sketch "Schizzo1" along normal blind 26 contours A28 L72 L73 L78 A33 L81 | L68 L72 L73 L78 L81 bodies 9 10 11
extrude "Estrusione74" add sketch "Schizzo1" along normal blind 1 separate body contours L49 L52 A20 A22 | L49 A20 A21 A22 A23 L108 | A20 A22 L108 L109 L110 | L51 L52 A20 A22 | L49 L50 A21 A23 | A21 A23 L108 L110 L111 | L51 A20 A21 A22 A23 L110 | L50 L51 A21 A23 | L57 L58 L59 L60 L85 | L60 L82 L83 L84 L85 picked at (258.7276, 240.2386) picked at (287.3942, 240.2386) makes body 12
extrude "Estrusione33" add sketch "Schizzo1" along normal blind 81.5 from surface at 1 contours L49 L52 A20 A22 | L51 L52 A20 A22 | L49 L50 A21 A23 | L50 L51 A21 A23 | L57 L58 L59 L60 L85 | L60 L82 L83 L84 L85 bodies 12
sketch "Foro display" plane through (0, 225.7386, 0) normal (0, -1, 0) x (1, 0, 0)
  line L0 (305.0609, 0) -> (305.0609, 82.5)
  line L1 (305.0609, 82.5) -> (215.0609, 82.5)
  circle A0 centre (273.0609, 41.75) radius 11
  line L2 (215.0609, 82.5) -> (215.0609, 0)
  line L3 (215.0609, 0) -> (305.0609, 0)
  line L4 (305.0609, 0) -> (241.0609, 0)
  line L5 (215.0609, 82.5) -> (305.0609, 82.5) construction
  line L6 (305.0609, 82.5) -> (305.0609, 0) construction
  line L7 (305.0609, 0) -> (215.0609, 0) construction
  line L8 (215.0609, 0) -> (215.0609, 82.5) construction
  dimension "d147" = 22
  dimension "d423" = 32
  dimension "d424" = 41.75
  constraint horizontal L5
  constraint vertical L6
  constraint horizontal L7
  constraint vertical L8
  constraint coincident L1.end L2.start
  constraint coincident L0.start L3.end
  measures "d147" diameter of A0
  measures "d423" distance of A0.centre L6
  measures "d424" distance of A0.centre L7
extrude "Estrusione34" cut sketch "Foro display" against normal blind 1.5 contours A0 bodies 12